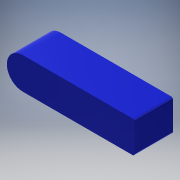
# Autodesk Inventor part: バッテリー(G6 HI-VOLTAGE 2400MAH 3S 80CMAX LIPO)
Saved by Autodesk Inventor 2018 (Build 220112000, 112)
## iProperties
Created: 2016-05-03
Part Number: バッテリー(G6 HI-VOLTAGE 2400MAH 3S 80CMAX LIPO)
Material: 一般
Document SubType Name: Modeling
Designer: hiroaki
Mass: 184 g
Surface Area: 139.6 cm^2
Volume: 87.9375 cm^3
Density: 2.0924 g/cm^3
Appearance: 青 - 壁塗料 - 光沢
Author: hiroaki
Autodesk Inventor part; units mm, degrees
ref_plane "YZ Plane" through (0, 0, 0) normal (1, 0, 0) x (0, 1, 0)
ref_plane "XZ Plane" through (0, 0, 0) normal (0, 1, 0) x (-1, 0, 0)
ref_plane "XY Plane" through (0, 0, 0) normal (0, 0, 1) x (1, 0, 0)
sketch "スケッチ1" plane through (0, 0, 0) normal (0, 0, 1) x (1, 0, 0)
  line L0 (-56.5, -17) -> (56.5, -17)
  line L1 (56.5, -17) -> (56.5, 17)
  line L2 (56.5, 17) -> (-56.5, 17)
  line L3 (-56.5, 17) -> (-56.5, -17)
  line L4 (-56.5, -17) -> (56.5, 17) construction
  line L5 (56.5, -17) -> (-56.5, 17) construction
  point P0 (0, 0)
  dimension "d0" = 113
  dimension "d1" = 34
  constraints: 12 end point, 2 midpoint, 2 parallel, 1 horizontal, 1 perpendicular
  measures "d0" distance of L1.end L2.end
  measures "d1" distance of L0.end L1.end
extrude "押し出し1" add sketch "スケッチ1" along normal blind 14
mirror "ミラー1" about plane through (0, 0, 0) normal (0, 0, -1) of "押し出し1"
fillet "フィレット1" radius 14 2 edges at (-56.5, 0, 14) (-56.5, 0, -14)
fillet "フィレット2" radius 2 2 edges at (56.5, 0, 14) (56.5, 0, -14)
